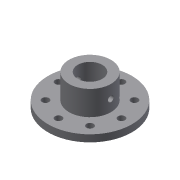
# Autodesk Inventor part: hub
Saved by Autodesk Inventor 2022 (Build 260148000, 148)
## iProperties
Created: 2005-10-20
Part Number: hub
Document SubType Name: Modeling
Designer: dchu
Density: 1 g/cm^3
Material: Generic
Appearance: Default
Author: dchu
Autodesk Inventor part; units mm, degrees
ref_plane "YZ Plane" through (0, 0, 0) normal (1, 0, 0) x (0, 1, 0)
ref_plane "XZ Plane" through (0, 0, 0) normal (0, 1, 0) x (-1, 0, 0)
sketch "Sketch2" plane through (0, 0, 0) normal (1, 0, 0) x (0, 1, 0)
  line L0 (0, 58.5) -> (0, -4.5) projected
  line L1 (-6, 0) -> (78, 0) projected
  line L2 (60, 0) -> (60, 10)
  line L3 (60, 10) -> (30, 10)
  line L4 (30, 10) -> (30, 45)
  line L5 (30, 45) -> (0, 45)
  line L6 (0, 0) -> (60, 0)
  line L7 (0, 45) -> (0, 0)
  dimension "d0" = 60
  dimension "d1" = 30
  dimension "d2" = 10
  dimension "d3" = 35
  constraints: 12 end point, 4 point on line, 3 perpendicular, 2 collinear, 1 parallel
  measures "d0" distance between parallel lines of L0 L2
  measures "d1" distance between parallel lines of L0 L4
  measures "d2" distance of L2.start L2.end
  measures "d3" distance of L3.end L4.end
revolve "Revolution1" add sketch "Sketch2" angle 360 about axis through (0, 0, 0) along (0, 0, -1)
hole "Hole1" at (0, 0, 45) direction (0, 0, -1) diameter 35 end through all
sketch "Sketch3" plane through (0, 0, 10) normal (0, 0, 1) x (1, 0, 0)
  line L0 (-72, 0) -> (96, 0) projected
  line L1 (0, 96) -> (0, -72) projected
  point P0 (45, 0)
  dimension "d14" = 45
  constraints: 1 point on line
  measures "d14" distance from line of L1 point (45, 0)
hole "Hole2" at (45, 0, 10) direction (0, 0, -1) diameter 10 end through all
pattern_circular "Circular Pattern1" count 8 over 360 about axis through (0, 0, -10) along (0, 0, 1) of "Hole2"
ref_plane "Work Plane1" through (30, 0, 45) normal (1, 0, 0) x (0, 0, -1)
sketch "Sketch4" plane through (30, 0, 45) normal (1, 0, 0) x (0, 0, -1)
  line L0 (-13.5, 0) -> (49.5, 0) projected
  line L1 (45, -72) -> (45, 96) projected
  line L2 (45, -60) -> (45, 60) projected
  line L3 (0, -30) -> (0, 30) projected
  point P0 (18.5, 0)
  dimension "d26" = 18.5
  constraints: 1 point on line
  measures "d26" distance from line of L3 point (18.5, 0)
hole "Hole3" at (30, 0, 26.5) direction (-1, 0, 0) diameter 8 end through all
body "Solid1"
